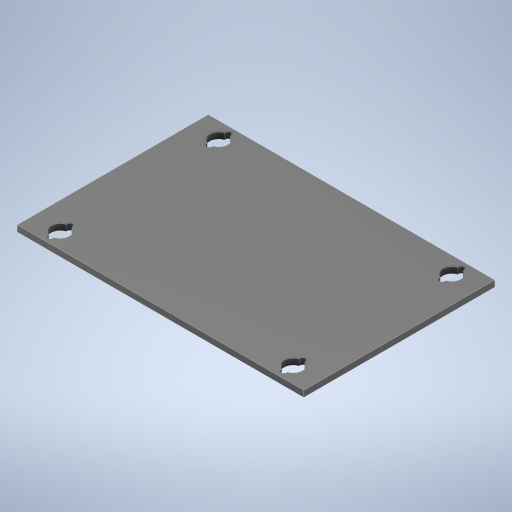
# Autodesk Inventor part: SUSTAINA-POWER-INPUT-BORAD
Saved by Autodesk Inventor 2024.2 (Build 282272000, 272)
## iProperties
Created: 2024-02-11
Part Number: SUSTAINA-POWER-INPUT-BORAD
Material: CFRP
Document SubType Name: Modeling
Designer: Masato Kubotera
Appearance: Smooth - Black
Vendor: JLCPCB
Surface Area: 78.5123 cm^2
Volume: 5.87025 cm^3
Author: Masato Kubotera
Autodesk Inventor part; units mm, degrees
ref_plane "YZ Plane" through (0, 0, 0) normal (1, 0, 0) x (0, 1, 0)
ref_plane "XZ Plane" through (0, 0, 0) normal (0, 1, 0) x (-1, 0, 0)
ref_plane "XY Plane" through (0, 0, 0) normal (0, 0, 1) x (1, 0, 0)
sketch "Sketch1" plane through (0, 0, 0) normal (0, 0, 1) x (1, 0, 0)
  line L0 (25, 37.5) -> (-25, 37.5)
  line L1 (-25, 37.5) -> (-25, -37.5)
  line L2 (-25, -37.5) -> (25, -37.5)
  line L3 (25, -37.5) -> (25, 37.5)
  line L4 (25, 37.5) -> (-25, -37.5) construction
  line L5 (-25, 37.5) -> (25, -37.5) construction
  line L6 (-20.75, -30.5) -> (20.75, -30.5) construction
  line L7 (20.75, -30.5) -> (20.75, 30.5) construction
  line L8 (20.75, 30.5) -> (-20.75, 30.5) construction
  line L9 (-20.75, 30.5) -> (-20.75, -30.5) construction
  line L10 (-20.75, -30.5) -> (20.75, 30.5) construction
  line L11 (20.75, -30.5) -> (-20.75, 30.5) construction
  circle A0 centre (20.75, 30.5) radius 2.4
  arc A1 (23.0395, 29.7801) -> (23.0395, 31.2199) centre (23.25, 30.5) ccw
  line L12 (0, 37.5) -> (0, -37.5) construction
  line L13 (25, 0) -> (-25, 0) construction
  circle A2 centre (20.75, -30.5) radius 2.4
  arc A3 (23.0395, -31.2199) -> (23.0395, -29.7801) centre (23.25, -30.5) ccw
  line L14 (0, -37.5) -> (0, 37.5) construction
  circle A4 centre (-20.75, 30.5) radius 2.4
  arc A5 (-23.0395, 31.2199) -> (-23.0395, 29.7801) centre (-23.25, 30.5) ccw
  circle A6 centre (-20.75, -30.5) radius 2.4
  arc A7 (-23.0395, -29.7801) -> (-23.0395, -31.2199) centre (-23.25, -30.5) ccw
  arc A8 (18.4605, 31.2199) -> (18.4605, 29.7801) centre (18.25, 30.5) ccw
  arc A9 (18.4605, -29.7801) -> (18.4605, -31.2199) centre (18.25, -30.5) ccw
  arc A10 (-18.4605, 29.7801) -> (-18.4605, 31.2199) centre (-18.25, 30.5) ccw
  arc A11 (-18.4605, -31.2199) -> (-18.4605, -29.7801) centre (-18.25, -30.5) ccw
  point P0 (0, 0)
  point P1 (24, 30.5)
  point P2 (17.5, 30.5)
  point P3 (18.4605, 29.7801)
  point P4 (18.4605, 31.2199)
  point P5 (18.4605, -31.2199)
  point P6 (18.4605, -29.7801)
  point P7 (-18.4605, -29.7801)
  point P8 (-18.4605, -31.2199)
  point P9 (-18.4605, 31.2199)
  point P10 (-18.4605, 29.7801)
  dimension "d0" = 50
  dimension "d1" = 75
  dimension "d2" = 4.8
  dimension "d4" = 1.5
  dimension "d6" = 14
  dimension "d9" = 61
  dimension "d10" = 41.5
  dimension "d11" = 6.5
  dimension "d12" = 1
  constraints: 30 end point, 26 point on circle, 26 symmetric about line, 12 centre point, 8 midpoint, 4 parallel, 2 horizontal, 2 perpendicular, 1 coincident, 1 point on line, 10 other
  measures "d0" distance of L2.end L1.end
  measures "d1" distance of L1.end L0.end
  measures "d2" diameter of A0
  measures "d4" diameter of A1
  measures "d6" diameter of L0 L8
  measures "d9" distance of L6.end L7.end
  measures "d10" distance of L7.end L8.end
  measures "d11" distance of point (24, 30.5) point (17.5, 30.5)
  measures "d12" distance from line of L3 point (24, 30.5)
extrude "Extrusion1" add sketch "Sketch1" along normal blind 1.6
body "Solid1"
